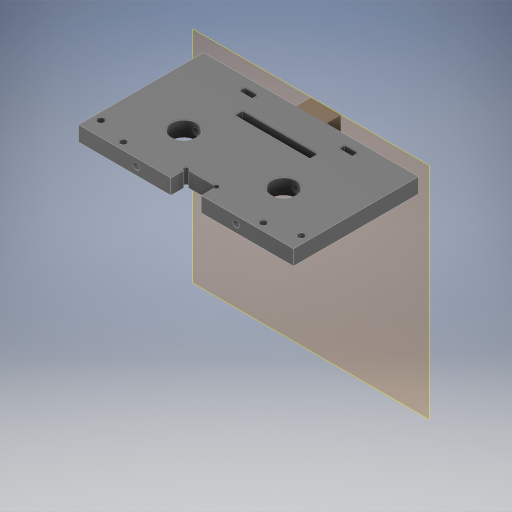
# Autodesk Inventor part: front of head
Saved by Autodesk Inventor 2024 (Build 280153000, 153)
## iProperties
Created: 2024-09-04
Part Number: front of head
Material: PMMA 플라스틱
Document SubType Name: Modeling
Designer: msi
Density: 1.188 g/cm^3
Appearance: 매끄러움 - 검은색
Mass: 21.4358 g
Surface Area: 100.054 cm^2
Volume: 21.4358 cm^3
Author: msi
Autodesk Inventor part; units mm, degrees
ref_plane "YZ Plane" through (0, 0, 0) normal (1, 0, 0) x (0, 1, 0)
ref_plane "XZ Plane" through (0, 0, 0) normal (0, 1, 0) x (-1, 0, 0)
ref_plane "XY Plane" through (0, 0, 0) normal (0, 0, 1) x (1, 0, 0)
ref_plane "작업 평면1" through (0, 0, 0) normal (0, 0, 1) x (1, 0, 0)
sketch "스케치1" plane through (0, 0, 0) normal (0, 0, 1) x (1, 0, 0)
  circle A0 centre (-20, 40) radius 1.35 projected
  circle A1 centre (20, 40) radius 1.35 projected
  line L0 (6.05, 36.95) -> (-6.05, 36.95) projected
  line L1 (-6.05, 36.95) -> (-6.05, 43.05) projected
  line L2 (-6.05, 43.05) -> (6.05, 43.05) projected
  line L3 (6.05, 43.05) -> (6.05, 36.95) projected
  line L4 (-37, 6) -> (-37, 45) projected
  line L5 (-37, 6) -> (-43, 6) projected
  line L6 (-43, 6) -> (-43, -6) projected
  line L7 (-43, -6) -> (-37, -6) projected
  line L8 (-37, -6) -> (-37, -35) projected
  line L9 (-37, -35) -> (37, -35) projected
  line L10 (37, -35) -> (37, -6) projected
  line L11 (37, -6) -> (43, -6) projected
  line L12 (43, -6) -> (43, 6) projected
  line L13 (43, 6) -> (37, 6) projected
  line L14 (37, 6) -> (37, 45) projected
  line L15 (-37, 45) -> (37, 45) projected
  circle A2 centre (-28.8, -30.8) radius 1.35 projected
  circle A3 centre (28.8, -30.8) radius 1.35 projected
  circle A4 centre (28.8, 30.8) radius 1.35 projected
  circle A5 centre (-20.8, -30.8) radius 1.6 projected
  circle A6 centre (-20.8, 30.8) radius 1.6 projected
  circle A7 centre (20.8, -30.8) radius 1.6 projected
  circle A8 centre (20.8, 30.8) radius 1.6 projected
  circle A9 centre (-28.8, 30.8) radius 1.35 projected
  line L16 (31.1, -8.4) -> (31.1, -13.6) projected
  line L17 (31.1, -13.6) -> (28.9, -13.6) projected
  line L18 (28.9, -13.6) -> (28.9, -8.4) projected
  line L19 (28.9, -8.4) -> (31.1, -8.4) projected
  line L20 (-31.1, -8.4) -> (-28.9, -8.4) projected
  line L21 (-28.9, -8.4) -> (-28.9, -13.6) projected
  line L22 (-28.9, -13.6) -> (-31.1, -13.6) projected
  line L23 (-31.1, -13.6) -> (-31.1, -8.4) projected
  line L24 (-31.1, 13.6) -> (-28.9, 13.6) projected
  line L25 (-28.9, 13.6) -> (-28.9, 8.4) projected
  line L26 (-28.9, 8.4) -> (-31.1, 8.4) projected
  line L27 (-31.1, 8.4) -> (-31.1, 13.6) projected
  line L28 (28.9, 13.6) -> (31.1, 13.6) projected
  line L29 (31.1, 13.6) -> (31.1, 8.4) projected
  line L30 (31.1, 8.4) -> (28.9, 8.4) projected
  line L31 (28.9, 8.4) -> (28.9, 13.6) projected
  line L32 (37, 37) -> (-37, 37)
  line L33 (-37, 37) -> (-37, 43)
  line L34 (-37, 43) -> (37, 43)
  line L35 (37, 43) -> (37, 37)
  line L36 (37, 37) -> (-37, 43) construction
  line L37 (-37, 37) -> (37, 43) construction
  point P0 (0, 0)
  point P1 (0, 40)
  dimension "d0" = 74
  dimension "d1" = 6
  constraints: 12 end point, 2 midpoint, 2 parallel, 1 horizontal, 1 perpendicular
  measures "d0" distance of L33.end L34.end
  measures "d1" distance of L32.end L33.end
extrude "돌출1" add sketch "스케치1" along normal blind 50 contours L32 L1 L34 L3 | L3 L34 L14 L32 | L32 L4 L34 L1
sketch "스케치2" plane through (0, 0, 50) normal (0, 0, 1) x (1, 0, 0)
  line L0 (6.05, 43) -> (-6.05, 43)
  line L1 (-6.05, 43) -> (-6.05, 37)
  line L2 (-6.05, 37) -> (6.05, 37)
  line L3 (6.05, 37) -> (6.05, 43)
  line L4 (6.05, 43) -> (-6.05, 37) construction
  line L5 (-6.05, 43) -> (6.05, 37) construction
  point P0 (0, 0)
  point P1 (0, 40)
  dimension "d4" = 12.1
  dimension "d5" = 6
  constraints: 12 end point, 2 midpoint, 2 parallel, 1 horizontal, 1 perpendicular
  measures "d4" distance of L2.end L1.end
  measures "d5" distance of L1.end L0.end
extrude "돌출2" cut sketch "스케치2" against normal blind 6.1
sketch "스케치3" plane through (0, 0, 0) normal (0, 0, -1) x (-1, 0, 0)
  line L0 (-6, 37) -> (6, 37)
  line L1 (6, 37) -> (6, 43)
  line L2 (6, 43) -> (-6, 43)
  line L3 (-6, 43) -> (-6, 37)
  line L4 (-6, 37) -> (6, 43) construction
  line L5 (6, 37) -> (-6, 43) construction
  point P0 (0, 0)
  point P1 (0, 40)
  dimension "d8" = 12
  dimension "d9" = 6
  constraints: 12 end point, 2 midpoint, 2 parallel, 1 horizontal, 1 perpendicular
  measures "d8" distance of L2.end L1.end
  measures "d9" distance of L1.end L0.end
extrude "돌출3" add sketch "스케치3" along normal blind 6
sketch "스케치4" plane through (37, 43, 50) normal (0, 1, 0) x (1, 0, 0)
  line L0 (-58.35, 0) -> (-58.35, 50) projected
  line L1 (-55.65, 0) -> (-55.65, 50) projected
  line L2 (-18.35, 0) -> (-18.35, 50) projected
  line L3 (-15.65, 0) -> (-15.65, 50) projected
  line L4 (-15.65, 35) -> (-18.35, 35)
  line L5 (-55.65, 35) -> (-58.35, 35)
  line L6 (-14.4, 36.1) -> (-19.6, 33.9) construction
  line L7 (-19.6, 36.1) -> (-14.4, 33.9) construction
  line L8 (-54.4, 36.1) -> (-59.6, 36.1)
  line L9 (-59.6, 36.1) -> (-59.6, 33.9)
  line L10 (-59.6, 33.9) -> (-54.4, 33.9)
  line L11 (-54.4, 33.9) -> (-54.4, 36.1)
  line L12 (-54.4, 36.1) -> (-59.6, 33.9) construction
  line L13 (-59.6, 36.1) -> (-54.4, 33.9) construction
  circle A0 centre (-9, 3) radius 1.35
  circle A1 centre (-65, 3) radius 1.35
  line L14 (-14.4, 46.1) -> (-19.6, 46.1)
  line L15 (-19.6, 46.1) -> (-19.6, 43.9)
  line L16 (-19.6, 43.9) -> (-14.4, 43.9)
  line L17 (-14.4, 43.9) -> (-14.4, 46.1)
  line L18 (-14.4, 46.1) -> (-19.6, 43.9) construction
  line L19 (-19.6, 46.1) -> (-14.4, 43.9) construction
  line L20 (-54.4, 46.1) -> (-59.6, 46.1)
  line L21 (-59.6, 46.1) -> (-59.6, 43.9)
  line L22 (-59.6, 43.9) -> (-54.4, 43.9)
  line L23 (-54.4, 43.9) -> (-54.4, 46.1)
  line L24 (-54.4, 46.1) -> (-59.6, 43.9) construction
  line L25 (-59.6, 46.1) -> (-54.4, 43.9) construction
  point P0 (-37, 50)
  point P1 (-17, 35)
  point P2 (-57, 35)
  point P3 (-17, 45)
  point P4 (-57, 45)
  dimension "d12" = 5.2
  dimension "d13" = 2.2
  dimension "d14" = 5.2
  dimension "d15" = 2.2
  dimension "d16" = 2.7
  dimension "d17" = 2.7
  dimension "d20" = 5.2
  dimension "d21" = 2.2
  dimension "d22" = 5.2
  dimension "d23" = 2.2
  constraints: 44 end point, 10 midpoint, 6 parallel, 5 horizontal, 4 point on line, 3 perpendicular, 2 centre point
  measures "d12" distance of L7.end L6.end
  measures "d13" distance of L6.end L7.start
  measures "d14" distance of L10.end L9.end
  measures "d15" distance of L9.end L8.end
  measures "d16" diameter of A0
  measures "d17" diameter of A1
  measures "d20" distance of L16.end L15.end
  measures "d21" distance of L15.end L14.end
  measures "d22" distance of L22.end L21.end
  measures "d23" distance of L21.end L20.end
extrude "돌출5" cut sketch "스케치4" against normal blind 50 contours L22 L21 L20 L0 | L0 L20 L1 L22 | L1 L20 L23 L22 | L16 L15 L14 L2 | L2 L14 L3 L16 | L3 L14 L17 L16 | A0 | A1
sketch "스케치5" plane through (-37, 37, 0) normal (-1, 0, 0) x (0, 0, 1)
  line L0 (50, 6) -> (0, 6)
  line L1 (0, 6) -> (0, 0)
  line L2 (0, 0) -> (50, 0)
  line L3 (50, 0) -> (50, 6)
  point P0 (0, -37)
  constraints: 8 end point, 2 parallel, 1 horizontal, 1 perpendicular
extrude "돌출6" add sketch "스케치5" along normal blind 6
sketch "스케치6" plane through (37, 37, 0) normal (1, 0, 0) x (0, 0, -1)
  line L0 (-50, 0) -> (0, 0)
  line L1 (0, 0) -> (0, 6)
  line L2 (0, 6) -> (-50, 6)
  line L3 (-50, 6) -> (-50, 0)
  point P0 (0, -37)
  dimension "d28" = 6
  constraints: 8 end point, 2 parallel, 1 horizontal, 1 perpendicular
  measures "d28" distance of L1.end L0.end
extrude "돌출7" add sketch "스케치6" along normal blind 6
sketch "스케치7" plane through (-6.05, 43, 43.9) normal (0, 1, 0) x (1, 0, 0)
  circle A0 centre (26.05, 13) radius 5
  circle A1 centre (-13.95, 13) radius 5
  line L0 (21.05, 28.5) -> (-8.95, 28.5)
  line L1 (-8.95, 28.5) -> (-8.95, 31.5)
  line L2 (-8.95, 31.5) -> (21.05, 31.5)
  line L3 (21.05, 31.5) -> (21.05, 28.5)
  line L4 (21.05, 28.5) -> (-8.95, 31.5) construction
  line L5 (-8.95, 28.5) -> (21.05, 31.5) construction
  point P0 (6.05, 43.9)
  point P1 (6.05, 30)
  dimension "d31" = 10
  dimension "d32" = 10
  dimension "d35" = 3
  constraints: 12 end point, 2 centre point, 2 midpoint, 2 parallel, 1 horizontal, 1 perpendicular
  measures "d31" diameter of A0
  measures "d32" diameter of A1
  measures "d35" distance of L0.end L1.end
extrude "돌출9" cut sketch "스케치7" against normal blind 10
sketch "스케치8" plane through (-6.05, 43, 43.9) normal (0, 1, 0) x (1, 0, 0)
  line L0 (-8.95, 28.5) -> (-8.95, 31.5) projected
  line L1 (-8.95, 31.5) -> (21.05, 31.5) projected
  line L2 (21.05, 31.5) -> (21.05, 28.5) projected
  line L3 (21.05, 28.5) -> (-8.95, 28.5) projected
  circle A0 centre (-13.95, 13) radius 5 projected
  circle A1 centre (26.05, 13) radius 5 projected
  circle A2 centre (-21.95, -3.1) radius 1.35 projected
  line L4 (-16.55, 37.8) -> (-16.55, 40) projected
  line L5 (-16.55, 40) -> (-11.35, 40) projected
  line L6 (-11.35, 40) -> (-11.35, 37.8) projected
  line L7 (-11.35, 37.8) -> (-16.55, 37.8) projected
  circle A3 centre (34.05, -3.1) radius 1.35 projected
  line L8 (23.45, 40) -> (28.65, 40) projected
  line L9 (28.65, 40) -> (28.65, 37.8) projected
  line L10 (28.65, 37.8) -> (23.45, 37.8) projected
  line L11 (23.45, 37.8) -> (23.45, 40) projected
  line L12 (0, -6.1) -> (0, 0) projected
  line L13 (0, 0) -> (12.1, 0) projected
  line L14 (12.1, 0) -> (12.1, -6.1) projected
  line L15 (12.1, -6.1) -> (49.05, -6.1) projected
  line L16 (49.05, 43.9) -> (49.05, -6.1) projected
  line L17 (12.05, 43.9) -> (49.05, 43.9) projected
  line L18 (12.05, 43.9) -> (12.05, 49.9) projected
  line L19 (0.05, 49.9) -> (12.05, 49.9) projected
  line L20 (0.05, 43.9) -> (0.05, 49.9) projected
  line L21 (0.05, 43.9) -> (-36.95, 43.9) projected
  line L22 (-36.95, -6.1) -> (-36.95, 43.9) projected
  line L23 (0, -6.1) -> (-36.95, -6.1) projected
  circle A4 centre (-33.95, -0.1) radius 1.35
  circle A5 centre (46.05, 0) radius 1.35
  point P0 (6.05, 43.9)
  dimension "d38" = 2.7
  dimension "d41" = 2.7
  constraints: 2 centre point
  measures "d38" diameter of A4
  measures "d41" diameter of A5
extrude "돌출11" cut sketch "스케치8" against normal blind 10 contours A4 | A5
sketch "스케치9" plane through (-6.05, 43, 43.9) normal (0, 1, 0) x (1, 0, 0)
  line L0 (0, 0) -> (12.1, 0) projected
  line L1 (12.1, 0) -> (12.1, -6.1) projected
  line L2 (0, -6.1) -> (0, 0) projected
  circle A0 centre (12.1, 0) radius 1
  circle A1 centre (0, 0) radius 1
  point P0 (6.05, 43.9)
  point P1 (12.1, -1)
  point P2 (11.1, 0)
  dimension "d44" = 2
  dimension "d45" = 2
  constraints: 2 centre point, 2 coincident
  measures "d44" diameter of A0
  measures "d45" diameter of A1
extrude "돌출12" cut sketch "스케치9" against normal blind 10 contours L2 A1 L0 | L0 A1 L2 | A0 L1 L0 picked at (11.443, 0.0798)
